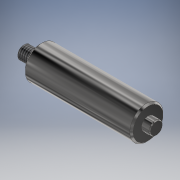
# Autodesk Inventor part: Albero cuscinetto
Saved by Autodesk Inventor 2018 (Build 220112000, 112)
## iProperties
Created: 2020-05-28
Part Number: Albero cuscinetto
Material: Generico
Document SubType Name: Modeling
Designer: Francesco
Density: 1 g/cm^3
Appearance: Acciaio - Lucido
Author: Francesco
Autodesk Inventor part; units mm, degrees
ref_plane "YZ Plane" through (0, 0, 0) normal (1, 0, 0) x (0, 1, 0)
ref_plane "XZ Plane" through (0, 0, 0) normal (0, 1, 0) x (-1, 0, 0)
ref_plane "XY Plane" through (0, 0, 0) normal (0, 0, 1) x (1, 0, 0)
sketch "Schizzo1" plane through (0, 0, 0) normal (0, 0, 1) x (1, 0, 0)
  line L0 (-42.5, 0) -> (42.5, 0)
  line L1 (-42.5, 0) -> (-42.5, 4)
  line L2 (-42.5, 4) -> (-32.5, 4)
  line L3 (-32.5, 4) -> (-32.5, 10)
  line L4 (-32.5, 10) -> (32.5, 10)
  line L5 (32.5, 10) -> (32.5, 4)
  line L6 (32.5, 4) -> (42.5, 4)
  line L7 (42.5, 4) -> (42.5, 0)
  point P0 (0, 0)
  point P1 (0, 0)
  point P2 (0, 10)
  dimension "d0" = 8
  dimension "d1" = 10
  dimension "d2" = 20
  dimension "d3" = 65
  dimension "d4" = 10
  constraints: 17 end point, 5 perpendicular, 2 coincident, 2 midpoint, 2 point on line, 1 horizontal, 1 vertical, 1 vertical alignment
  measures "d0" diameter of L2 L0
  measures "d1" distance between parallel lines of L3 L1
  measures "d2" diameter of L4 L0
  measures "d3" distance of L3.end L4.end
  measures "d4" distance between parallel lines of L5 L7
revolve "Rivoluzione1" add sketch "Schizzo1" angle 360 about axis through (-42.5, 0, 0) along (1, 0, 0)
chamfer "Smusso1" distance 0.5 angle 45 2 edges at (-42.5, -4, 0) (42.5, -4, 0)
thread "Filettatura1" size "M8x1.25" class "6g" standard "ISO Metric profile" full length
chamfer "Smusso2" distance 1 angle 45 2 edges at (-32.5, -10, 0) (32.5, -10, 0)
